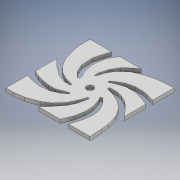
# Autodesk Inventor part: LOGO
Saved by Autodesk Inventor 2018 (Build 220112000, 112)
## iProperties
Created: 2017-06-07
Part Number: LOGO
Material: Generic
Document SubType Name: Modeling
Designer: Soichi
Density: 1 g/cm^3
Appearance: Default
Author: Soichi
Autodesk Inventor part; units mm, degrees
ref_plane "YZ Plane" through (0, 0, 0) normal (1, 0, 0) x (0, 1, 0)
ref_plane "XZ Plane" through (0, 0, 0) normal (0, 1, 0) x (-1, 0, 0)
ref_plane "XY Plane" through (0, 0, 0) normal (0, 0, 1) x (1, 0, 0)
sketch "Sketch2" plane through (0, 0, 0) normal (0, 0, 1) x (1, 0, 0)
  line L0 (112.918, 112.918) -> (93.1579, 111.5065)
  line L1 (93.1579, 111.5065) -> (76.9264, 107.6251)
  line L2 (76.9264, 107.6251) -> (65.2821, 102.3322)
  line L3 (65.2821, 102.3322) -> (54.6964, 93.1579)
  line L4 (54.6964, 93.1579) -> (49.7564, 84.6893)
  line L5 (49.7564, 84.6893) -> (46.2278, 74.1036)
  line L6 (46.2278, 74.1036) -> (45.0731, 74.1036)
  line L7 (45.0731, 74.1036) -> (45.0731, 79.4331)
  line L8 (45.0731, 79.4331) -> (48.1403, 90.6879)
  line L9 (48.1403, 90.6879) -> (53.786, 100.2151)
  line L10 (53.786, 100.2151) -> (61.9018, 107.978)
  line L11 (61.9018, 107.978) -> (68.9589, 112.918)
  line L12 (68.9589, 112.918) -> (39.8993, 112.918)
  line L13 (39.8993, 112.918) -> (33.795, 101.9794)
  line L14 (33.795, 101.9794) -> (31.325, 90.6879)
  line L15 (31.325, 90.6879) -> (31.325, 82.1768)
  line L16 (31.325, 82.1768) -> (33.4422, 73.045)
  line L17 (33.4422, 73.045) -> (38.0293, 63.165)
  line L18 (38.0293, 63.165) -> (38.0293, 60.3406)
  line L19 (38.0293, 60.3406) -> (35.351, 60.3406)
  line L20 (35.351, 60.3406) -> (28.3539, 68.105)
  line L21 (28.3539, 68.105) -> (24.1196, 77.985)
  line L22 (24.1196, 77.985) -> (23.4139, 93.5108)
  line L23 (23.4139, 93.5108) -> (29.0596, 112.918)
  line L24 (29.0596, 112.918) -> (0, 112.918)
  line L25 (0, 112.918) -> (0, 98.7833)
  line L26 (0, 98.7833) -> (2.2424, 86.4536)
  line L27 (2.2424, 86.4536) -> (6.4767, 73.3979)
  line L28 (6.4767, 73.3979) -> (13.181, 62.4593)
  line L29 (13.181, 62.4593) -> (20.5911, 55.755)
  line L30 (20.5911, 55.755) -> (29.7654, 50.8149)
  line L31 (29.7654, 50.8149) -> (39.9982, 48.3449)
  line L32 (39.9982, 48.3449) -> (39.9982, 46.4407)
  line L33 (39.9982, 46.4407) -> (31.2895, 46.4407)
  line L34 (31.2895, 46.4407) -> (21.5243, 50.1092)
  line L35 (21.5243, 50.1092) -> (9.5272, 58.9307)
  line L36 (9.5272, 58.9307) -> (0, 68.4578)
  line L37 (0, 68.4578) -> (0, 39.3982)
  line L38 (0, 39.3982) -> (8.1157, 35.65)
  line L39 (8.1157, 35.65) -> (16.5843, 33.18)
  line L40 (16.5843, 33.18) -> (25.4058, 31.7686)
  line L41 (25.4058, 31.7686) -> (34.6869, 31.7686)
  line L42 (34.6869, 31.7686) -> (47.283, 36.7086)
  line L43 (47.283, 36.7086) -> (49.2864, 36.7086)
  line L44 (49.2864, 36.7086) -> (49.2864, 35.1999)
  line L45 (49.2864, 35.1999) -> (41.6373, 29.7654)
  line L46 (41.6373, 29.7654) -> (32.1101, 25.8839)
  line L47 (32.1101, 25.8839) -> (18.3486, 24.8253)
  line L48 (18.3486, 24.8253) -> (5.9986, 27.2954)
  line L49 (5.9986, 27.2954) -> (0, 29.0596)
  line L50 (0, 29.0596) -> (0, 0)
  line L51 (0, 0) -> (10.4465, 0)
  line L52 (10.4465, 0) -> (22.9358, 1.6695)
  line L53 (22.9358, 1.6695) -> (39.1673, 7.3152)
  line L54 (39.1673, 7.3152) -> (48.6944, 13.3138)
  line L55 (48.6944, 13.3138) -> (57.5159, 23.1938)
  line L56 (57.5159, 23.1938) -> (62.8088, 33.7796)
  line L57 (62.8088, 33.7796) -> (66.3373, 43.6596)
  line L58 (66.3373, 43.6596) -> (68.5691, 43.6596)
  line L59 (68.5691, 43.6596) -> (67.6027, 37.7558)
  line L60 (67.6027, 37.7558) -> (65.4856, 28.9344)
  line L61 (65.4856, 28.9344) -> (60.8984, 20.1129)
  line L62 (60.8984, 20.1129) -> (52.7827, 9.88)
  line L63 (52.7827, 9.88) -> (43.9613, 0)
  line L64 (43.9613, 0) -> (73.0209, 0)
  line L65 (73.0209, 0) -> (78.5105, 13.7615)
  line L66 (78.5105, 13.7615) -> (80.6276, 24.7001)
  line L67 (80.6276, 24.7001) -> (80.6276, 35.1817)
  line L68 (80.6276, 35.1817) -> (77.099, 46.9301)
  line L69 (77.099, 46.9301) -> (74.629, 51.5173)
  line L70 (74.629, 51.5173) -> (74.629, 53.0196)
  line L71 (74.629, 53.0196) -> (77.3682, 53.0196)
  line L72 (77.3682, 53.0196) -> (83.1526, 46.9301)
  line L73 (83.1526, 46.9301) -> (87.7398, 39.1673)
  line L74 (87.7398, 39.1673) -> (89.5041, 33.1687)
  line L75 (89.5041, 33.1687) -> (90.2098, 26.1115)
  line L76 (90.2098, 26.1115) -> (88.7983, 15.5258)
  line L77 (88.7983, 15.5258) -> (87.3869, 9.5272)
  line L78 (87.3869, 9.5272) -> (83.8583, 0)
  line L79 (83.8583, 0) -> (112.918, 0)
  line L80 (112.918, 0) -> (112.1296, 16.5843)
  line L81 (112.1296, 16.5843) -> (110.7181, 27.5229)
  line L82 (110.7181, 27.5229) -> (106.8367, 40.5787)
  line L83 (106.8367, 40.5787) -> (99.7795, 51.5173)
  line L84 (99.7795, 51.5173) -> (90.9581, 58.9273)
  line L85 (90.9581, 58.9273) -> (78.608, 64.573)
  line L86 (78.608, 64.573) -> (69.4337, 67.043)
  line L87 (69.4337, 67.043) -> (69.4337, 69.8808)
  line L88 (69.4337, 69.8808) -> (79.8223, 69.8808)
  line L89 (79.8223, 69.8808) -> (87.5122, 67.9309)
  line L90 (87.5122, 67.9309) -> (95.2751, 64.0494)
  line L91 (95.2751, 64.0494) -> (101.6265, 58.7566)
  line L92 (101.6265, 58.7566) -> (107.6251, 52.4051)
  line L93 (107.6251, 52.4051) -> (112.918, 45.7008)
  line L94 (112.918, 45.7008) -> (112.918, 74.7605)
  line L95 (112.918, 74.7605) -> (103.0379, 78.9217)
  line L96 (103.0379, 78.9217) -> (91.3936, 81.7445)
  line L97 (91.3936, 81.7445) -> (79.6057, 81.7445)
  line L98 (79.6057, 81.7445) -> (69.8693, 78.5688)
  line L99 (69.8693, 78.5688) -> (62.8121, 75.3931)
  line L100 (62.8121, 75.3931) -> (61.5243, 75.3931)
  line L101 (61.5243, 75.3931) -> (61.5243, 77.0169)
  line L102 (61.5243, 77.0169) -> (66.3407, 80.6826)
  line L103 (66.3407, 80.6826) -> (75.1622, 85.6226)
  line L104 (75.1622, 85.6226) -> (85.395, 88.0926)
  line L105 (85.395, 88.0926) -> (95.3458, 88.0926)
  line L106 (95.3458, 88.0926) -> (101.9794, 87.034)
  line L107 (101.9794, 87.034) -> (112.918, 83.8583)
  line L108 (112.918, 83.8583) -> (112.918, 112.918)
  circle A0 centre (56.459, 56.459) radius 4.5706
  line L109 (112.918, 0) -> (0, 112.918) construction
  line L110 (0, 0) -> (112.918, 0) construction
  line L111 (112.918, 0) -> (112.918, 112.918) construction
  line L112 (112.918, 112.918) -> (0, 112.918) construction
  line L113 (0, 112.918) -> (0, 0) construction
  dimension "d15" = 29.0597
  dimension "d16" = 29.0597
  dimension "d17" = 29.0597
  dimension "d18" = 29.0597
  dimension "d19" = 29.0597
  dimension "d20" = 29.0597
  dimension "d21" = 29.0597
  dimension "d22" = 29.0597
  dimension "d23" = 112.918
  dimension "d24" = 112.918
  dimension "d25" = 112.918
  dimension "d26" = 112.918
  dimension "d27" = 112.918
  dimension "d28" = 112.918
  constraints: 228 end point, 7 collinear, 3 horizontal, 2 coincident, 2 parallel, 1 centre point, 1 midpoint, 1 perpendicular, 1 vertical
  measures "d15" distance of L23.end L24.end
  measures "d16" distance of L107.end L0.start
  measures "d17" distance of L78.end L79.end
  measures "d18" distance of L63.end L64.end
  measures "d19" distance of L49.end L50.end
  measures "d20" distance of L11.end L12.end
  measures "d21" distance of L93.end L94.end
  measures "d22" distance of L36.end L37.end
  measures "d23" distance of L0.start L24.end
  measures "d24" distance of L79.end L0.start
  measures "d25" distance of point (0, 0) L79.end
  measures "d26" distance of L24.end point (0, 0)
  measures "d27" distance of L111.end L112.end
  measures "d28" distance of L110.end L111.end
extrude "Extrusion1" add sketch "Sketch2" along normal blind 5
equation "\"d16\" = d15"
equation "\"d17\" = d15"
equation "\"d18\" = d15"
equation "\"d19\" = d15"
equation "\"d20\" = d15"
equation "\"d21\" = d20"
equation "\"d22\" = d15"
equation "\"d24\" = d23"
equation "\"d25\" = d23"
equation "\"d26\" = d23"
equation "\"d27\" = d23"
equation "\"d28\" = d23"
body "Solid1"
